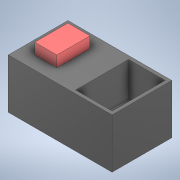
# Autodesk Inventor part: Разъем220
Saved by Autodesk Inventor 2020 (Build 240168000, 168)
## iProperties
Created: 2020-05-06
Part Number: Разъем220
Material: Типовые
Document SubType Name: Modeling
Designer: Михаил
Density: 1 g/cm^3
Appearance: По умолчанию
Author: Михаил
Autodesk Inventor part; units mm, degrees
ref_plane "YZ Plane" through (0, 0, 0) normal (1, 0, 0) x (0, 1, 0)
ref_plane "XZ Plane" through (0, 0, 0) normal (0, 1, 0) x (-1, 0, 0)
ref_plane "XY Plane" through (0, 0, 0) normal (0, 0, 1) x (1, 0, 0)
sketch "Эскиз1" plane through (0, 0, 0) normal (0, 1, 0) x (-1, 0, 0)
  line L0 (0, 0) -> (47, 0)
  line L1 (47, 0) -> (47, -27)
  line L2 (47, -27) -> (0, -27)
  line L3 (0, -27) -> (0, 0)
  dimension "d0" = 47
  dimension "d1" = 27
  constraints: 8 end point, 2 parallel, 1 horizontal, 1 perpendicular
  measures "d0" distance of L1.end L2.end
  measures "d1" distance of L0.end L1.end
extrude "Выдавливание1" add sketch "Эскиз1" along normal blind 22.5
sketch "Эскиз2" plane through (0, 22.5, 0) normal (0, 1, 0) x (1, 0, 0)
  line L0 (-18, 1.5) -> (-1.5, 1.5)
  line L1 (-1.5, 1.5) -> (-1.5, 25.5)
  line L2 (-1.5, 25.5) -> (-18, 25.5)
  line L3 (-18, 25.5) -> (-18, 1.5)
  line L4 (-47, 0) -> (0, 0) projected
  line L5 (0, 0) -> (0, 27) projected
  dimension "d4" = 16.5
  dimension "d5" = 24
  dimension "d6" = 1.5
  dimension "d7" = 1.5
  constraints: 8 end point, 2 parallel, 1 horizontal, 1 perpendicular
  measures "d4" distance of L2.end L1.end
  measures "d5" distance of L1.end L0.end
  measures "d6" distance between parallel lines of L4 L0
  measures "d7" distance between parallel lines of L5 L1
extrude "Выдавливание2" cut sketch "Эскиз2" against normal blind 15.5
sketch "Эскиз3" plane through (0, 22.5, 0) normal (0, 1, 0) x (1, 0, 0)
  line L0 (-41, 6) -> (-31, 6)
  line L1 (-31, 6) -> (-31, 21)
  line L2 (-31, 21) -> (-41, 21)
  line L3 (-41, 21) -> (-41, 6)
  line L4 (-47, 27) -> (-47, 0) projected
  line L5 (-47, 0) -> (0, 0) projected
  dimension "d10" = 10
  dimension "d11" = 15
  dimension "d12" = 6
  dimension "d13" = 6
  constraints: 8 end point, 2 parallel, 1 horizontal, 1 perpendicular
  measures "d10" distance of L2.end L1.end
  measures "d11" distance of L1.end L0.end
  measures "d12" distance between parallel lines of L4 L3
  measures "d13" distance between parallel lines of L5 L0
extrude "Выдавливание3" add sketch "Эскиз3" along normal blind 5
